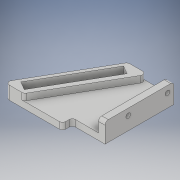
# Autodesk Inventor part: PhoneStandRight
Saved by Autodesk Inventor 2019 (Build 230136000, 136)
## iProperties
Created: 2019-10-11
Part Number: PhoneStandRight
Material: Generic
Document SubType Name: Modeling
Designer: james
Density: 1 g/cm^3
Appearance: Default
Author: james
Autodesk Inventor part; units mm, degrees
ref_plane "YZ Plane" through (0, 0, 0) normal (1, 0, 0) x (0, 1, 0)
ref_plane "XZ Plane" through (0, 0, 0) normal (0, 1, 0) x (-1, 0, 0)
ref_plane "XY Plane" through (0, 0, 0) normal (0, 0, 1) x (1, 0, 0)
sketch "Sketch1" plane through (0, 0, 0) normal (0, 1, 0) x (-1, 0, 0)
  line L0 (47.3286, 48.1428) -> (-41.5714, 48.1428)
  line L1 (-41.5714, 48.1428) -> (-41.5714, -28.2969)
  line L2 (-41.5714, -28.2969) -> (3.1961, -28.2969)
  line L3 (47.3286, 48.1428) -> (3.1961, -28.2969)
  point P0 (0, 0)
  dimension "d0" = 60
  dimension "d1" = 88.265
  dimension "d2" = 88.9
  constraints: 8 end point, 1 horizontal, 1 parallel, 1 perpendicular
  measures "d0" angle of L0 L3
  measures "d1" distance of L2.end L0.start
  measures "d2" distance of L0.start L0.end
extrude "Extrusion1" add sketch "Sketch1" along normal blind 6.35
sketch "Sketch2" plane through (41.5714, 0, 48.1428) normal (1, 0, 0) x (0, 0, -1)
  line L0 (0, 19.05) -> (76.4397, 19.05)
  line L1 (76.4397, 19.05) -> (76.4397, -12.7)
  line L2 (76.4397, -12.7) -> (0, -12.7)
  line L3 (0, -12.7) -> (0, 19.05)
  line L4 (0, 0) -> (76.4397, 0) projected
  line L5 (0, 6.35) -> (76.4397, 6.35) projected
  line L6 (0, 0) -> (0, 6.35) projected
  line L7 (76.4397, 0) -> (76.4397, 6.35) projected
  point P0 (48.1428, 0)
  dimension "d5" = 12.7
  dimension "d6" = 12.7
  dimension "d7" = 0
  dimension "d8" = 0
  constraints: 8 end point, 2 parallel, 1 horizontal, 1 perpendicular
  measures "d5" distance between parallel lines of L2 L4
  measures "d6" distance between parallel lines of L5 L0
  measures "d7" distance between parallel lines of L6 L3
  measures "d8" distance between parallel lines of L7 L1
extrude "Extrusion2" add sketch "Sketch2" against normal blind 6.35 contours L0 L1 L5 L3 | L4 L1 L2 L3
sketch "Sketch3" plane through (0, 6.35, 0) normal (0, 1, 0) x (1, 0, 0)
  line L0 (-47.3286, -48.1428) -> (35.2214, -48.1428) projected
  line L1 (-3.1961, 28.2969) -> (-47.3286, -48.1428) projected
  line L2 (35.2214, 28.2969) -> (-3.1961, 28.2969) projected
  line L3 (-47.3286, -48.1428) -> (35.2214, -48.1428) projected
  line L4 (-47.3286, -48.1428) -> (-3.1961, 28.2969)
  line L5 (-3.1961, 28.2969) -> (16.4546, 28.2969)
  line L6 (35.2214, 28.2969) -> (-3.1961, 28.2969) projected
  line L7 (16.4546, 28.2969) -> (-27.6779, -48.1428)
  line L8 (-47.3286, -48.1428) -> (-27.6779, -48.1428)
  dimension "d13" = 17.018
  constraints: 8 end point, 2 point on line, 1 horizontal, 1 parallel
  measures "d13" distance between parallel lines of L7 L1
extrude "Extrusion3" add sketch "Sketch3" along normal blind 6.35
sketch "Sketch4" plane through (0, 12.7, 0) normal (0, 1, 0) x (1, 0, 0)
  line L0 (-3.1961, 28.2969) -> (-47.3286, -48.1428) projected
  line L1 (-38.9235, -39.9348) -> (-2.411, 23.3067)
  line L2 (-2.411, 23.3067) -> (5.7279, 18.6077)
  line L3 (5.7279, 18.6077) -> (-30.7846, -44.6338)
  line L4 (-30.7846, -44.6338) -> (-38.9235, -39.9348)
  point P0 (0, 0)
  dimension "d16" = 9.398
  dimension "d17" = 3.175
  dimension "d18" = 73.025
  constraints: 8 end point, 3 perpendicular
  measures "d16" distance of L3.end L1.start
  measures "d17" distance between parallel lines of L0 L1
  measures "d18" distance of L2.end L3.end
extrude "Extrusion4" cut sketch "Sketch4" against normal blind 25.4
sketch "Sketch5" plane through (41.5714, 19.05, 48.1428) normal (1, 0, 0) x (0, 0, -1)
  line L0 (76.4397, -31.75) -> (0, -31.75) projected
  line L1 (76.4397, -31.75) -> (76.4397, 0) projected
  line L2 (0, 0) -> (76.4397, 0) projected
  point P0 (48.1428, -19.05)
  point P1 (70.0897, -6.35)
  point P2 (31.9897, -6.35)
  dimension "d22" = 0
  dimension "d23" = 6.35
  dimension "d24" = 38.1
  dimension "d48" = 6.35
  measures "d22" vertical distance of point (31.99, -6.35) point (70.09, -6.35)
  measures "d23" distance from line of L1 point (70.09, -6.35)
  measures "d24" distance of point (31.99, -6.35) point (70.09, -6.35)
  measures "d48" distance from line of point (70.09, -6.35) L2
hole "Hole1" at (41.5714, 12.7, -21.9469) at (41.5714, 12.7, 16.1531) direction (-1, 0, 0) diameter 4.4958 depth 25.4 tip angle 118.188 clearance for "Flat Head Machine Screw (82)" size "#8" standard "Ansi Unified Screw Threads"
fillet "Fillet1" radius 3.175 1 edges at (-47.3286, 6.35, 48.1428)
fillet "Fillet2" radius 3.175 1 edges at (-3.1961, 6.35, -28.2969)
fillet "Fillet4" radius 3.175 6 edges at (38.3964, -12.7, -28.2969) (38.3964, -12.7, 48.1428) (38.3964, 19.05, -28.2969) (38.3964, 19.05, 48.1428) (16.4546, 9.525, -28.2969) (-27.6779, 9.525, 48.1428)
sketch "Sketch8" plane through (41.5714, -12.7, 44.9678) normal (1, 0, 0) x (0, 0, -1)
  line L0 (-49.5788, 45.5329) -> (6.35, 45.5329)
  line L1 (6.35, 45.5329) -> (6.35, -8.6732)
  line L2 (6.35, -8.6732) -> (-49.5788, -8.6732)
  line L3 (-49.5788, -8.6732) -> (-49.5788, 45.5329)
  line L4 (-3.175, 3.175) -> (-3.175, 28.575) projected
  point P0 (44.9678, 12.7)
  dimension "d41" = 9.525
  constraints: 8 end point, 2 parallel, 1 horizontal, 1 perpendicular
  measures "d41" distance between parallel lines of L4 L1
extrude "Extrusion7" cut sketch "Sketch8" against normal blind 31.75
fillet "Fillet5" radius 3.175 1 edges at (9.8214, 3.175, 48.1428)
fillet "Fillet6" radius 3.175 2 edges at (38.3964, 19.05, 38.6178) (38.3964, -12.7, 38.6178)
fillet "Fillet7" radius 3.175 1 edges at (9.8214, 3.175, 38.6178)
sketch "Sketch10" plane through (41.5714, -9.525, -28.2969) normal (1, 0, 0) x (0, 0, -1)
  line L0 (-71.5248, -9.7742) -> (12.1423, -9.7742)
  line L1 (12.1423, -9.7742) -> (12.1423, 9.525)
  line L2 (12.1423, 9.525) -> (-71.5248, 9.525)
  line L3 (-71.5248, 9.525) -> (-71.5248, -9.7742)
  line L4 (0, 9.525) -> (-66.9147, 9.525) projected
  point P0 (-28.2969, 9.525)
  dimension "d49" = 0
  constraints: 8 end point, 2 parallel, 1 horizontal, 1 perpendicular
  measures "d49" distance between parallel lines of L2 L4
extrude "Extrusion8" cut sketch "Sketch10" against normal blind 31.75
sketch "Sketch11" plane through (0, 0, 0) normal (0, -1, 0) x (1, 0, 0)
  point P0 (0, 0)
  point P1 (7.8072, -24.9207)
  point P2 (-39.4342, 44.6338)
hole "Hole2" at (7.8072, 0, -24.9207) at (-39.4342, 0, 44.6338) direction (0, 1, 0) diameter 2.6416 depth 10.9728 tip angle 118.188 thread size "6-32 UNC" class "2B" standard "ANSI Unified Screw Threads"
body "Solid1"
